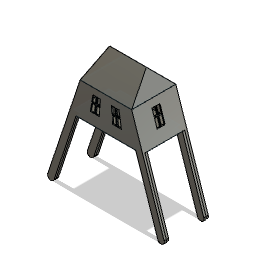
form10 v5 (Autodesk Fusion 360 design; units mm, degrees)
Autodesk Fusion 360 part; units mm, degrees
note: some values were not read from the file. Chosen so that the rebuilt part matches the saved one: which bodies a step acts on; which face or edge a step refers to. Set by a fixed rule: which sketch regions a step uses.
(part 1 of 2)
sketch "Sketch1" plane through (0, 0, 0) normal (0, 0, 1) x (1, 0, 0)
  line L0 (-100, 300) -> (100, 300)
  line L1 (100, 300) -> (100, 500)
  line L2 (100, 500) -> (-100, 500)
  line L3 (-100, 500) -> (-100, 300)
  line L4 (0, 0) -> (200, 0)
  line L5 (200, 0) -> (0, 0)
  line L6 (0, 0) -> (-200, 0)
  line L7 (-200, 0) -> (-100, 300)
  line L8 (100, 300) -> (200, 0)
  line L9 (-100, 500) -> (-266.666667, 0)
  line L10 (100, 500) -> (266.666667, 0)
  line L11 (163.504389, 309.486833) -> (135.04389, 300)
  line L12 (135.04389, 300) -> (100, 300)
  line L13 (-163.504389, 309.486833) -> (-135.04389, 300)
  line L14 (-135.04389, 300) -> (-100, 300)
  line L15 (-135.04389, 300) -> (-235.04389, 0)
  line L16 (135.04389, 300) -> (235.04389, 0)
  line L17 (266.666667, 0) -> (235.04389, 0)
  line L18 (-235.04389, 0) -> (-266.666667, 0)
  dimension "d1" = 200
  dimension "d2" = 200
  dimension "d3" = 30
  dimension "d4" = 30
  constraint horizontal L0
  constraint vertical L1
  constraint horizontal L2
  constraint vertical L3
  constraint coincident L4.start L5.end
  constraint perpendicular L3 L4
  constraint perpendicular L3 L6
  constraint parallel L7 L9
  constraint parallel L8 L10
  constraint perpendicular L10 L11
  constraint perpendicular L9 L13
  constraint parallel L9 L15
  constraint parallel L10 L16
  measures "d1" distance of L0.start L0.end
  measures "d2" distance of L0.start L2.end
extrude "Extrude1" add sketch "Sketch1" along normal blind 200 contours L0 L1 L2 L3 | L3 L9 L13 L14 | L1 L10 L11 L12 | L9 L13 L15 L18 | L10 L11 L16 L17 picked at (-33.333333, 433.333333) picked at (-121.16813, 369.828944) picked at (121.16813, 369.828944) picked at (-221.738315, 103.162278) picked at (221.738315, 103.162278) makes body 1
sketch "Sketch2" plane through (0, 0, 0) normal (1, 0, 0) x (0, 0, -1)
  line L0 (0, 500) -> (-200, 500)
  line L1 (-200, 500) -> (-200, 400)
  line L2 (-200, 400) -> (0, 400)
  line L3 (0, 400) -> (0, 500)
  line L4 (-100, 500) -> (0, 400)
  line L5 (-100, 500) -> (-200, 400)
  constraint horizontal L0
  constraint vertical L1
  constraint horizontal L2
  constraint vertical L3
  constraint midpoint L0 L4.start
  constraint perpendicular L4 L5
sketch "Sketch3" plane through (0, 500, 0) normal (0, 1, 0) x (-1, 0, 0)
  line L0 (-100, 0) -> (100, 0)
  line L1 (100, 0) -> (100, 200)
  line L2 (100, 200) -> (-100, 200)
  line L3 (-100, 200) -> (-100, 0)
sketch "Sketch4" plane through (0, 0, 0) normal (0, 0, -1) x (-1, 0, 0)
  line L0 (-135.04389, 300) -> (135.04389, 300)
  line L1 (135.04389, 300) -> (235.04389, 0)
  line L2 (235.04389, 0) -> (266.666667, 0)
  line L3 (266.666667, 0) -> (100, 500)
  line L4 (100, 500) -> (-100, 500)
  line L5 (-100, 500) -> (-266.666667, 0)
  line L6 (-266.666667, 0) -> (-235.04389, 0)
  line L7 (-235.04389, 0) -> (-135.04389, 300)
  line L8 (0, 500) -> (0, 550)
  line L9 (100, 550) -> (-100, 550)
  line L10 (100, 500) -> (83.333333, 550)
  line L11 (-100, 500) -> (-83.333333, 550)
  point P0 (0, 500)
  dimension "d7" = 50
  constraint coincident P0 L8.start
  constraint perpendicular L4 L8
  constraint horizontal L9
  constraint coincident L3.end L4.start
  constraint parallel L3 L10
  constraint coincident L4.end L5.start
  constraint parallel L5 L11
  measures "d7" distance of P0 L8.end
extrude "Extrude2" add sketch "Sketch4" against normal blind 200 contours L4 L8 L9 L11 | L4 L8 L9 L10 picked at (-61.111111, 516.666667) picked at (61.111111, 516.666667) bodies 1
sketch "Sketch5" plane through (0, 0, 0) normal (1, 0, 0) x (0, 0, -1)
  line L0 (-200, 550) -> (0, 550)
  line L1 (0, 550) -> (0, 450)
  line L2 (0, 450) -> (-200, 450)
  line L3 (-200, 450) -> (-200, 550)
  line L4 (-200, 550) -> (0, 550)
  line L5 (0, 550) -> (0, 500)
  line L6 (0, 500) -> (-200, 500)
  line L7 (-200, 500) -> (-200, 550)
  line L8 (-100, 550) -> (-200, 500)
  line L9 (0, 500) -> (-100, 550)
  line L10 (0, 450) -> (-100, 550)
  line L11 (-200, 450) -> (-100, 550)
  constraint horizontal L0
  constraint vertical L1
  constraint horizontal L2
  constraint vertical L3
  constraint horizontal L4
  constraint vertical L5
  constraint horizontal L6
  constraint vertical L7
  constraint midpoint L1 L5.end
  constraint midpoint L4 L8.start
  constraint perpendicular L10 L11
extrude "Extrude3" cut sketch "Sketch5" along normal blind 200 and the other way blind 200 contours L0 L3 L4 L7 L8 | L0 L1 L4 L5 L9 picked at (-166.666667, 533.333333) picked at (-33.333333, 533.333333) bodies 1
sketch "Sketch6" plane through (0, 0, 0) normal (1, 0, 0) x (0, 0, -1)
  line L0 (-20, 0) -> (-180, 0)
  line L1 (-180, 0) -> (-180, 300)
  line L2 (-180, 300) -> (-20, 300)
  line L3 (-20, 300) -> (-20, 0)
  dimension "d14" = 160
  dimension "d15" = 300
  constraint horizontal L0
  constraint vertical L1
  constraint horizontal L2
  constraint vertical L3
  measures "d14" distance of L0.start L0.end
  measures "d15" distance of L0.start L2.end
extrude "Extrude4" cut sketch "Sketch6" along normal blind 430 and the other way blind 320 bodies 1
sketch "Sketch7" plane through (0, 0, 0) normal (0, 0, -1) x (-1, 0, 0)
  line L0 (100, 500) -> (-100, 500)
  line L1 (-100, 500) -> (-266.666667, 0)
  line L2 (-266.666667, 0) -> (-235.04389, 0)
  line L3 (-235.04389, 0) -> (-135.04389, 300)
  line L4 (-135.04389, 300) -> (135.04389, 300)
  line L5 (135.04389, 300) -> (235.04389, 0)
  line L6 (235.04389, 0) -> (266.666667, 0)
  line L7 (266.666667, 0) -> (100, 500)
  line L8 (235.04389, 0) -> (263.504389, 9.486833)
  line L9 (249.27414, 4.743416) -> (240.606216, 30.747187)
  circle A0 centre (249.27414, 4.743416) radius 15
  line L10 (263.504389, 9.486833) -> (266.666667, 0)
  constraint perpendicular L7 L8
  constraint perpendicular L8 L9
extrude "Extrude5" cut sketch "Sketch7" against normal blind 300 contours L6 L7 A0 L10 picked at (264.700479, 0.516842) bodies 1
extrude "Extrude6" add sketch "Sketch7" against normal blind 20 separate body contours L6 L8 A0 | L8 L9 A0 | L8 L9 A0 | L6 A0 picked at (249.27414, 1.581139) picked at (248.203436, 14.660304) picked at (241.078294, 10.428413) picked at (245.376265, -2.550327) makes body 2
copy_body "CopyPasteBodies1" bodies 2 makes body 3
move_body "Move1" bodies 3 to x (1, 0, 0) y (0, 1, 0) z (0, 0, 1) at (0, 0, 180)
copy_body "CopyPasteBodies2" bodies 3 makes body 4
sketch "Sketch8" plane through (0, 0, 0) normal (0, 0, -1) x (-1, 0, 0)
  line L0 (-100, 500) -> (-266.666667, 0)
  line L1 (-235.04389, 0) -> (-263.504389, 9.486833)
  line L2 (-249.27414, 4.743416) -> (-238.791899, 36.190138)
  circle A0 centre (-249.27414, 4.743416) radius 15
  line L3 (-263.504389, 0) -> (-266.666667, 0)
  line L4 (-263.504389, 9.486833) -> (-266.666667, 0)
  point P0 (-235.04389, 0)
  constraint perpendicular L0 L1
  constraint perpendicular L1 L2
extrude "Extrude7" cut sketch "Sketch8" against normal blind 3000 contours L0 A0 L3 L4 picked at (-264.722183, 0.621872) bodies 1
extrude "Extrude8" add sketch "Sketch8" against normal blind 20 separate body contours L1 L2 A0 | L1 A0 | L1 L2 A0 picked at (-256.067662, 12.046781) picked at (-255.959942, -2.656664) picked at (-242.065982, 11.639917) makes body 5
copy_body "CopyPasteBodies3" bodies 5 makes body 6
move_body "Move2" bodies 6 to x (1, 0, 0) y (0, 1, 0) z (0, 0, 1) at (0, 0, 180)
extrude "Extrude9" cut sketch "Sketch5" along normal blind 225 and the other way blind 225 contours L0 L3 L4 L7 L8 | L6 L8 L11 | L0 L1 L4 L5 L9 | L6 L9 L10 | L3 L6 L11 | L1 L6 L10 picked at (-166.666667, 533.333333) picked at (-150, 516.666667) picked at (-33.333333, 533.333333) picked at (-50, 516.666667) picked at (-183.333333, 483.333333) picked at (-16.666667, 483.333333) bodies 1
sketch "Sketch9" plane through (0, 0, 200) normal (0, 0, 1) x (1, 0, 0)
  line L0 (116.666667, 450) -> (-116.666667, 450)
  line L1 (-116.666667, 450) -> (-263.504389, 9.486833)
  arc A0 (-263.504389, 9.486833) -> (-263.504389, 0) centre (-249.27414, 4.743416) ccw
  line L2 (-263.504389, 0) -> (-235.04389, 0)
  line L3 (-235.04389, 0) -> (-135.04389, 300)
  line L4 (-135.04389, 300) -> (135.04389, 300)
  line L5 (135.04389, 300) -> (235.04389, 0)
  line L6 (235.04389, 0) -> (263.504389, 0)
  arc A1 (263.504389, 0) -> (263.504389, 9.486833) centre (249.27414, 4.743416) ccw
  line L7 (263.504389, 9.486833) -> (116.666667, 450)
  line L8 (116.666667, 450) -> (-10.364311, 831.092932)
  line L9 (-116.666667, 450) -> (23.051535, 869.154604)
  line L10 (0, 800) -> (49.840939, -0.317043)
  line L11 (49.840939, -0.317043) -> (-46.807566, -0.317043)
  line L12 (-46.807566, -0.317043) -> (-150, -0.317043)
  line L13 (-150, -0.317043) -> (0, 800)
  line L14 (49.840939, -0.317043) -> (150, -0.317043)
  line L15 (150, -0.317043) -> (0, 800)
  line L16 (-50, -0.317043) -> (-50, -20)
  line L17 (49.840939, -0.317043) -> (-50, -0.317043)
  line L18 (-50, -0.317043) -> (0, 800)
  line L19 (-125, 325) -> (125, 325)
  line L20 (125, 325) -> (125, 425)
  line L21 (125, 425) -> (-125, 425)
  line L22 (-125, 425) -> (-125, 325)
  line L23 (-125, 375) -> (125, 375)
  line L24 (-98.403783, -0.317043) -> (0, 800)
  line L25 (99.92047, -0.317043) -> (0, 800)
  line L26 (-100.388834, -0.072969) -> (-0.015179, 816.265027)
  line L27 (101.905062, -0.069264) -> (-0.015179, 816.265027)
  line L28 (-96.418732, -0.561117) -> (0.015179, 783.734974)
  line L29 (97.935878, -0.564821) -> (0.015179, 783.734974)
  line L30 (-125, 373) -> (125, 373)
  line L31 (-125, 377) -> (125, 377)
  line L32 (-145.180647, 3.682957) -> (0, 778.286596)
  line L33 (145.180647, 3.682957) -> (0, 778.286596)
  line L34 (49.840939, 3.682957) -> (145.180647, 3.682957)
  line L35 (49.840939, 3.682957) -> (-46.807566, 3.682957)
  line L36 (-46.807566, 3.682957) -> (-145.180647, 3.682957)
  line L37 (-53.992216, -0.067628) -> (0.00636, 864.251996)
  line L38 (0.00636, 864.251996) -> (53.833205, -0.068418)
  line L39 (-121, 329) -> (121, 329)
  line L40 (121, 329) -> (121, 421)
  line L41 (121, 421) -> (-121, 421)
  line L42 (-121, 421) -> (-121, 329)
  line L43 (116.666667, 450, 0) -> (116.666667, 450, -200)
  line L44 (-116.666667, 450, 0) -> (-116.666667, 450, -200)
  line L45 (-170, 300) -> (170, 300)
  line L46 (170, 300) -> (170, 450)
  line L47 (170, 450) -> (-170, 450)
  line L48 (-170, 450) -> (-170, 300)
  line L49 (0, 300) -> (167.029465, 300)
  line L50 (167.029465, 300) -> (167.029465, 450)
  line L51 (167.029465, 450) -> (0, 450)
  line L52 (0, 450) -> (0, 300)
  point P0 (116.666667, 450)
  point P1 (-116.666667, 450)
  dimension "d32" = 2
  dimension "d33" = -2
  dimension "d34" = 2
  dimension "d35" = -2
  dimension "d36" = 4
  dimension "d37" = -4
  dimension "d38" = -4
  constraint parallel L7 L8
  constraint parallel L1 L9
  constraint coincident L8 L10.start
  constraint coincident L9 L10.start
  constraint horizontal L11
  constraint parallel L11 L12
  constraint parallel L11 L14
  constraint horizontal L19
  constraint vertical L20
  constraint horizontal L21
  constraint vertical L22
  constraint coincident L7 L20.end
  constraint midpoint L22 L23.start
  constraint midpoint L20 L23.end
  constraint horizontal L45
  constraint vertical L46
  constraint horizontal L47
  constraint vertical L48
  constraint horizontal L49
  constraint vertical L50
  constraint horizontal L51
  constraint vertical L52
sketch "Sketch10" plane through (0, 0, 200) normal (0, 0, 1) x (1, 0, 0)
  line L0 (0, 300) -> (-166.775998, 300)
  line L1 (-166.775998, 300) -> (-166.775998, 450.114505)
  line L2 (0, 450.114505) -> (0, 300)
  line L3 (116.666667, 450) -> (83.333333, 550)
  line L4 (83.333333, 550) -> (-18.03309, 854.099269)
  line L5 (-116.666667, 450) -> (-83.333333, 550)
  line L6 (-83.333333, 550) -> (27.18713, 881.561391)
  line L7 (30, 350) -> (70, 350)
  line L8 (-30, 350) -> (-70, 350)
  line L9 (-70, 350) -> (0, 800)
  line L10 (70, 350) -> (0, 800)
  line L11 (30, 350) -> (0, 800)
  line L12 (-30, 350) -> (0, 800)
  line L13 (59.111111, 420) -> (-59.111111, 420)
  line L14 (50, 350) -> (0, 800)
  line L15 (-50, 350) -> (0, 800)
  line L16 (-25.333333, 420) -> (-70, 350)
  line L17 (-59.111111, 420) -> (-30, 350)
  line L18 (59.111111, 420) -> (30, 350)
  line L19 (25.333333, 420) -> (70, 350)
  line L20 (45.783133, 387.951807) -> (-45.783133, 387.951807)
  line L21 (45.783133, 387.951807) -> (64.096386, 387.951807)
  line L22 (-45.783133, 387.951807) -> (-64.096386, 387.951807)
  line L23 (-45.783133, 389.951807) -> (-64.096386, 389.951807)
  line L24 (45.783133, 389.951807) -> (-45.783133, 389.951807)
  line L25 (45.783133, 389.951807) -> (64.096386, 389.951807)
  line L26 (-45.783133, 385.951807) -> (-64.096386, 385.951807)
  line L27 (45.783133, 385.951807) -> (-45.783133, 385.951807)
  line L28 (45.783133, 385.951807) -> (64.096386, 385.951807)
  line L29 (-51.987767, 350.220863) -> (0, 818.11077)
  line L30 (51.987767, 350.220863) -> (0, 818.11077)
  line L31 (-48.012233, 349.779137) -> (0, 781.88923)
  line L32 (48.012233, 349.779137) -> (0, 781.88923)
  line L33 (-51.987767, 350.220863) -> (-53.194502, 339.36025)
  line L34 (51.987767, 350.220863) -> (53.06275, 340.546021)
  line L35 (-64.096386, 385.951807) -> (-76.613224, 385.951807)
  line L36 (64.096386, 385.951807) -> (88.42743, 385.951807)
  point P0 (-83.333333, 550)
  point P1 (-116.666667, 450)
  point P2 (116.666667, 450)
  point P3 (83.333333, 550)
  dimension "d40" = 2
  dimension "d41" = -2
  dimension "d42" = 2
  dimension "d43" = -2
  constraint horizontal L0
  constraint vertical L1
  constraint vertical L2
  constraint parallel L3 L4
  constraint parallel L5 L6
  constraint horizontal L7
  constraint horizontal L8
  constraint coincident L6 L9.end
  constraint coincident L4 L9.end
  constraint midpoint L7 L14.start
  constraint midpoint L8 L15.start
  constraint horizontal L21
  constraint parallel L20 L22
  constraint parallel L29 L33
  constraint parallel L30 L34
  constraint parallel L26 L35
  constraint parallel L28 L36
extrude "Extrude10" cut sketch "Sketch10" against normal blind 340 contours L11 L19 L24 L32 | L13 L19 L32 | L13 L16 L31 | L12 L16 L24 L31 | L11 L18 L27 L32 | L12 L17 L27 L31 | L13 L18 L30 | L13 L17 L29 | L7 L18 L32 | L8 L17 L31 | L9 L17 L23 L29 | L10 L18 L25 L30 | L10 L19 L28 L30 L36 | L7 L19 L30 L34 | L8 L16 L29 L33 | L9 L16 L26 L29 L35 picked at (32.005474, 400.57405) picked at (36.296597, 410.590114) picked at (-36.296597, 410.590114) picked at (-32.005474, 400.57405) picked at (33.932773, 373.361693) picked at (-33.932773, 373.361693) picked at (50.238933, 410.590114) picked at (-50.238933, 410.590114) picked at (40.7276, 361.377757) picked at (-40.7276, 361.377757) picked at (-56.755848, 400.57405) picked at (56.755848, 400.57405) picked at (60.772036, 373.361693) picked at (56.73583, 361.451378) picked at (-56.73583, 361.451378) picked at (-60.772036, 373.361693) bodies 1
sketch "Sketch11" plane through (0, 0, 0) normal (1, 0, 0) x (0, 0, -1)
sketch "Sketch12" plane through (0, 0, 0) normal (1, 0, 0) x (0, 0, -1)
  line L0 (-105, 420) -> (-85, 420)
  line L1 (-85, 420) -> (-85, 350.000005)
  line L2 (-85, 350.000005) -> (-105, 350.000005)
  line L3 (-105, 350.000005) -> (-105, 420)
  line L4 (-105, 420) -> (-125, 420)
  line L5 (-125, 420) -> (-125, 350)
  line L6 (-125, 350) -> (-105, 350)
  line L7 (-105, 350) -> (-105, 420)
  line L8 (-103, 418) -> (-87, 418)
  line L9 (-87, 418) -> (-87, 352.000005)
  line L10 (-87, 352.000005) -> (-103, 352.000005)
  line L11 (-103, 352.000005) -> (-103, 418)
  line L12 (-107, 418) -> (-123, 418)
  line L13 (-123, 418) -> (-123, 352)
  line L14 (-123, 352) -> (-107, 352)
  line L15 (-107, 352) -> (-107, 418)
  line L16 (-107, 420) -> (-107, 350)
  line L17 (-103, 420) -> (-103, 350)
  line L18 (-87, 420) -> (-87, 350)
  line L19 (-123, 420) -> (-123, 350)
  line L20 (-85, 390) -> (-125, 390)
  line L21 (-125, 386.000006) -> (-85, 386.000006)
  dimension "d46" = 20
  dimension "d47" = 70
  dimension "d48" = 2
  dimension "d49" = -2
  constraint horizontal L0
  constraint vertical L1
  constraint horizontal L2
  constraint vertical L3
  constraint horizontal L4
  constraint vertical L5
  constraint horizontal L6
  constraint vertical L7
  constraint coincident L4 L16.start
  constraint coincident L6 L16.end
  constraint perpendicular L6 L16
  constraint coincident L0 L17.start
  constraint coincident L2 L17.end
  constraint perpendicular L2 L17
  constraint coincident L0 L18.start
  constraint coincident L2 L18.end
  constraint perpendicular L2 L18
  constraint coincident L4 L19.start
  constraint coincident L6 L19.end
  constraint perpendicular L6 L19
  constraint coincident L1 L20.start
  constraint coincident L5 L20.end
  constraint perpendicular L5 L20
  constraint perpendicular L1 L21
  measures "d46" distance of L0.start L0.end
  measures "d47" distance of L0.start L6.end
extrude "Extrude11" cut sketch "Sketch12" along normal blind 310 and the other way blind 250 contours L0 L8 L17 L18 | L4 L12 L16 L19 | L8 L9 L11 L17 L18 L20 | L12 L13 L15 L16 L19 L20 | L13 L14 L15 L16 L19 L21 | L9 L10 L11 L17 L18 L21 | L2 L10 L17 L18 | L6 L14 L16 L19 picked at (-97.666667, 418.666667) picked at (-117.666667, 418.666667) picked at (-97.666667, 408.666667) picked at (-117.666667, 408.666667) picked at (-112.333333, 363.333335) picked at (-97.666667, 363.333339) picked at (-92.333333, 351.333339) picked at (-117.666667, 350.666668) bodies 1
sketch "Sketch13" plane through (0, 0, 200) normal (0, 0, 1) x (1, 0, 0)
  line L0 (27.336546, 389.951807) -> (25.333333, 420)
  line L1 (25.333333, 420) -> (40.209914, 420)
  line L2 (40.209914, 420) -> (43.548602, 389.951807)
  line L3 (43.548602, 389.951807) -> (27.336546, 389.951807)
  line L4 (-63.785274, 389.951807) -> (-59.111111, 420)
  line L5 (-59.111111, 420) -> (-44.23453, 420)
  line L6 (-44.23453, 420) -> (-47.573218, 389.951807)
  line L7 (-47.573218, 389.951807) -> (-63.785274, 389.951807)
  line L8 (-64.407497, 385.951807) -> (-48.017663, 385.951807)
  line L9 (-48.017663, 385.951807) -> (-52.012308, 350)
  line L10 (-52.012308, 350) -> (-70, 350)
  line L11 (-70, 350) -> (-64.407497, 385.951807)
  line L12 (59.111111, 420) -> (63.785274, 389.951807)
  line L13 (63.785274, 389.951807) -> (47.573218, 389.951807)
  line L14 (47.573218, 389.951807) -> (44.23453, 420)
  line L15 (44.23453, 420) -> (59.111111, 420)
  line L16 (43.993047, 385.951807) -> (47.987692, 350)
  line L17 (47.987692, 350) -> (30, 350)
  line L18 (30, 350) -> (27.603213, 385.951807)
  line L19 (27.603213, 385.951807) -> (43.993047, 385.951807)
  line L20 (-43.548602, 389.951807) -> (-40.209914, 420)
  line L21 (-40.209914, 420) -> (-25.333333, 420)
  line L22 (-25.333333, 420) -> (-27.336546, 389.951807)
  line L23 (-27.336546, 389.951807) -> (-43.548602, 389.951807)
  line L24 (-47.987692, 350) -> (-43.993047, 385.951807)
  line L25 (-43.993047, 385.951807) -> (-27.603213, 385.951807)
  line L26 (-27.603213, 385.951807) -> (-30, 350)
  line L27 (-30, 350) -> (-47.987692, 350)
  line L28 (70, 350) -> (52.012308, 350)
  line L29 (52.012308, 350) -> (48.017663, 385.951807)
  line L30 (48.017663, 385.951807) -> (64.407497, 385.951807)
  line L31 (64.407497, 385.951807) -> (70, 350)
  line L32 (116.666667, 450) -> (-116.666667, 450)
  line L33 (-116.666667, 450) -> (-263.504389, 9.486833)
  arc A0 (-263.504389, 9.486833) -> (-263.504389, 0) centre (-249.27414, 4.743416) ccw
  line L34 (-263.504389, 0) -> (-235.04389, 0)
  line L35 (-235.04389, 0) -> (-135.04389, 300)
  line L36 (-135.04389, 300) -> (135.04389, 300)
  line L37 (135.04389, 300) -> (235.04389, 0)
  line L38 (235.04389, 0) -> (263.504389, 0)
  arc A1 (263.504389, 0) -> (263.504389, 9.486833) centre (249.27414, 4.743416) ccw
  line L39 (263.504389, 9.486833) -> (116.666667, 450)
  line L40 (200, 450) -> (-200, 450)
  line L41 (-200, 450) -> (-200, 602.828066)
  line L42 (-200, 602.828066) -> (200, 602.828066)
  line L43 (200, 602.828066) -> (200, 450)
  dimension "d54" = 400
  constraint horizontal L40
  constraint vertical L41
  constraint horizontal L42
  constraint vertical L43
  measures "d54" distance of L40.start L40.end
split "Split1" by curves path "Sketch13" along L42 L43 L40 L41 bodies 1 makes body 7 at (-45.01463, 300, 73.333333)
sketch "Sketch14" plane through (0, 325, 325) normal (0, 0.707107, 0.707107) x (1, 0, 0)
  line L0 (116.666667, 176.776695) -> (83.333333, 318.198052)
  line L1 (83.333333, 318.198052) -> (-83.333333, 318.198052)
  line L2 (-83.333333, 318.198052) -> (-116.666667, 176.776695)
  line L3 (-116.666667, 176.776695) -> (116.666667, 176.776695)
  line L4 (-79.374833, 313.198052) -> (-110.351144, 181.776695)
  line L5 (-110.351144, 181.776695) -> (110.351144, 181.776695)
  line L6 (110.351144, 181.776695) -> (79.374833, 313.198052)
  line L7 (79.374833, 313.198052) -> (-79.374833, 313.198052)
  dimension "d55" = -5
extrude "Extrude12" cut sketch "Sketch14" along normal blind -240 and the other way blind 5 contours L4 L5 L6 L7 picked at (-26.458278, 225.583814) bodies 1
sketch "Sketch15" plane through (0, 225, -225) normal (0, 0.707107, -0.707107) x (-1, 0, 0)
  line L0 (-83.333333, 459.619408) -> (-116.666667, 318.198052)
  line L1 (-116.666667, 318.198052) -> (116.666667, 318.198052)
  line L2 (116.666667, 318.198052) -> (83.333333, 459.619408)
  line L3 (83.333333, 459.619408) -> (-83.333333, 459.619408)
  line L4 (110.351144, 323.198052) -> (79.374833, 454.619408)
  line L5 (79.374833, 454.619408) -> (-79.374833, 454.619408)
  line L6 (-79.374833, 454.619408) -> (-110.351144, 323.198052)
  line L7 (-110.351144, 323.198052) -> (110.351144, 323.198052)
  dimension "d60" = -5
extrude "Extrude13" cut sketch "Sketch15" along normal blind -180 and the other way blind 5 contours L4 L5 L6 L7 picked at (26.458278, 367.00517) bodies 1
sketch "Sketch16" plane through (-240, 80, 0) normal (-0.948683, 0.316228, 0) x (0, 0, 1)
  line L0 (0, 390.014245) -> (200, 390.014245)
  line L1 (200, 390.014245) -> (100, 495.4235)
  line L2 (100, 495.4235) -> (0, 390.014245)
  line L3 (11.635441, 395.014245) -> (188.364559, 395.014245)
  line L4 (188.364559, 395.014245) -> (100, 488.158669)
  line L5 (100, 488.158669) -> (11.635441, 395.014245)
  line L6 (11.635441, 395.014245) -> (-12.394431, 369.684536)
  line L7 (188.364559, 395.014245) -> (205.575241, 376.872594)
  dimension "d65" = -5
  constraint parallel L5 L6
  constraint parallel L4 L7
extrude "Extrude14" cut sketch "Sketch16" along normal blind -40 and the other way blind 6 contours L0 L3 L6 L7 | L3 L4 L5 picked at (129.454853, 391.680911) picked at (100, 426.062386) bodies 1
sketch "Sketch17" plane through (240, 80, 0) normal (0.948683, 0.316228, 0) x (0, 0, -1)
  line L0 (-200, 390.014245) -> (0, 390.014245)
  line L1 (0, 390.014245) -> (-100, 495.4235)
  line L2 (-100, 495.4235) -> (-200, 390.014245)
  line L3 (-100, 490) -> (-7, 392.000006)
  line L4 (-7, 392.000006) -> (-0.785722, 386.104624)
  line L5 (-100, 490) -> (-193.000003, 392.000006)
  line L6 (-193.000003, 392.000006) -> (-201.192859, 383.366675)
  constraint perpendicular L2 L4
  constraint parallel L5 L6
extrude "Extrude15" cut sketch "Sketch17" along normal blind -50 and the other way blind 6 contours L0 L3 L4 L5 L6 picked at (-100.000001, 424.666671) bodies 1
sketch "Sketch18" plane through (-240, 80, 0) normal (-0.948683, 0.316228, 0) x (0, 0, 1)
  line L0 (0, 390.014245) -> (200, 390.014245)
  line L1 (200, 390.014245) -> (100, 495.4235)
  line L2 (100, 495.4235) -> (0, 390.014245)
  line L3 (100, 490) -> (7.077367, 392.050945)
  line L4 (7.077367, 392.050945) -> (-0.940246, 383.599639)
  line L5 (100, 490) -> (196.278995, 388.513028)
  line L6 (196.278995, 388.513028) -> (-0.940246, 383.599639)
  constraint parallel L2 L3
  constraint parallel L1 L5
extrude "Extrude16" cut sketch "Sketch18" along normal blind -40 and the other way blind 6 contours L0 L3 L4 L5 picked at (100.644061, 424.02173) bodies 1
sketch "Sketch19" plane through (0, 0, 0) normal (0, 0, -1) x (-1, 0, 0)
  line L0 (-25.333333, 420) -> (-27.336546, 389.951807)
  line L1 (-27.336546, 389.951807) -> (-43.548602, 389.951807)
  line L2 (-43.548602, 389.951807) -> (-40.209914, 420)
  line L3 (-40.209914, 420) -> (-25.333333, 420)
  line L4 (59.111111, 420) -> (63.785274, 389.951807)
  line L5 (63.785274, 389.951807) -> (47.573218, 389.951807)
  line L6 (47.573218, 389.951807) -> (44.23453, 420)
  line L7 (44.23453, 420) -> (59.111111, 420)
  line L8 (48.017663, 385.951807) -> (64.407497, 385.951807)
  line L9 (64.407497, 385.951807) -> (70, 350)
  line L10 (70, 350) -> (52.012308, 350)
  line L11 (52.012308, 350) -> (48.017663, 385.951807)
  line L12 (-63.785274, 389.951807) -> (-59.111111, 420)
  line L13 (-59.111111, 420) -> (-44.23453, 420)
  line L14 (-44.23453, 420) -> (-47.573218, 389.951807)
  line L15 (-47.573218, 389.951807) -> (-63.785274, 389.951807)
  line L16 (-47.987692, 350) -> (-43.993047, 385.951807)
  line L17 (-43.993047, 385.951807) -> (-27.603213, 385.951807)
  line L18 (-27.603213, 385.951807) -> (-30, 350)
  line L19 (-30, 350) -> (-47.987692, 350)
  line L20 (40.209914, 420) -> (43.548602, 389.951807)
  line L21 (43.548602, 389.951807) -> (27.336546, 389.951807)
  line L22 (27.336546, 389.951807) -> (25.333333, 420)
  line L23 (25.333333, 420) -> (40.209914, 420)
  line L24 (43.993047, 385.951807) -> (47.987692, 350)
  line L25 (47.987692, 350) -> (30, 350)
  line L26 (30, 350) -> (27.603213, 385.951807)
  line L27 (27.603213, 385.951807) -> (43.993047, 385.951807)
  line L28 (-52.012308, 350) -> (-70, 350)
  line L29 (-70, 350) -> (-64.407497, 385.951807)
  line L30 (-64.407497, 385.951807) -> (-48.017663, 385.951807)
  line L31 (-48.017663, 385.951807) -> (-52.012308, 350)
  line L32 (116.666667, 450) -> (-116.666667, 450)
  line L33 (-116.666667, 450) -> (-263.504389, 9.486833)
  arc A0 (-263.504389, 9.486833) -> (-263.504389, 0) centre (-249.27414, 4.743416) ccw
  line L34 (-263.504389, 0) -> (-235.04389, 0)
  line L35 (-235.04389, 0) -> (-135.04389, 300)
  line L36 (-135.04389, 300) -> (135.04389, 300)
  line L37 (135.04389, 300) -> (235.04389, 0)
  line L38 (235.04389, 0) -> (263.504389, 0)
  arc A1 (263.504389, 0) -> (263.504389, 9.486833) centre (249.27414, 4.743416) ccw
  line L39 (263.504389, 9.486833) -> (116.666667, 450)
  line L40 (-116.666667, 450) -> (-166.778531, 299.664408)
  line L41 (166.778531, 299.664408) -> (116.666667, 450)
  arc A2 (-258.760973, 7.905694) -> (-259.270847, 5) centre (-249.27414, 4.743416) ccw
  line L42 (-259.270847, 5) -> (-238.647686, 5)
  line L43 (-238.647686, 5) -> (-138.647686, 305)
  line L44 (-138.647686, 305) -> (138.647686, 305)
  line L45 (138.647686, 305) -> (238.647686, 5)
  line L46 (238.647686, 5) -> (259.270847, 5)
  arc A3 (259.270847, 5) -> (258.760973, 7.905694) centre (249.27414, 4.743416) ccw
  line L47 (258.760973, 7.905694) -> (113.062871, 445)
  line L48 (113.062871, 445) -> (-113.062871, 445)
  line L49 (-113.062871, 445) -> (-258.760973, 7.905694)
  line L50 (-138.647686, 305) -> (-176.025835, 305)
  line L51 (-176.025835, 305) -> (138.647686, 305)
  line L52 (210, 305) -> (138.647686, 305)
  dimension "d78" = -5
  constraint parallel L33 L40
  constraint parallel L39 L41
  constraint parallel L44 L50
  constraint parallel L51 L52
extrude "Extrude17" cut sketch "Sketch19" along normal blind -195 and the other way blind 5 contours L44 L47 L48 L49 L50 L51 L52 picked at (107.236852, 366.666667) bodies 7
sketch "Sketch20" plane through (0, 450, 0) normal (0, 1, 0) x (-1, 0, 0)
  line L0 (-116.666667, 0) -> (116.666667, 0)
  line L1 (116.666667, 0) -> (116.666667, 200)
  line L2 (116.666667, 200) -> (-116.666667, 200)
  line L3 (-116.666667, 200) -> (-116.666667, 0)
  line L4 (111.666667, 195) -> (-111.666667, 195)
  line L5 (-111.666667, 195) -> (-111.666667, 5)
  line L6 (-111.666667, 5) -> (111.666667, 5)
  line L7 (111.666667, 5) -> (111.666667, 195)
  dimension "d83" = -5
extrude "Extrude18" cut sketch "Sketch20" against normal blind 40 contours L4 L5 L6 L7 picked at (37.222222, 68.333333) bodies 7
sketch "Sketch21" plane through (0, 450, 0) normal (0, 1, 0) x (-1, 0, 0)
  line L0 (-111.666667, 195) -> (111.666667, 195)
  line L1 (111.666667, 195) -> (111.666667, 5)
  line L2 (111.666667, 5) -> (-111.666667, 5)
  line L3 (-111.666667, 5) -> (-111.666667, 195)
  line L4 (-116.666667, 0) -> (116.666667, 0)
  line L5 (116.666667, 0) -> (116.666667, 200)
  line L6 (116.666667, 200) -> (-116.666667, 200)
  line L7 (-116.666667, 200) -> (-116.666667, 0)
sketch "Sketch22" plane through (0, 450, 0) normal (0, 1, 0) x (-1, 0, 0)
  line L0 (-110.666667, 6) -> (110.666667, 6)
  line L1 (110.666667, 6) -> (110.666667, 194)
  line L2 (110.666667, 194) -> (-110.666667, 194)
  line L3 (-110.666667, 194) -> (-110.666667, 6)
  line L4 (-105.666667, 189) -> (-105.666667, 11)
  line L5 (-105.666667, 11) -> (105.666667, 11)
  line L6 (105.666667, 11) -> (105.666667, 189)
  line L7 (105.666667, 189) -> (-105.666667, 189)
  point P0 (-110.666667, 6)
  point P1 (110.666667, 194)
  dimension "d87" = -5
  constraint horizontal L0
  constraint vertical L1
  constraint horizontal L2
  constraint vertical L3
extrude "Extrude19" add sketch "Sketch22" along normal blind 2 and the other way blind 4 bodies 1
sketch "Sketch23" plane through (0, 300, 0) normal (0, -1, 0) x (1, 0, 0)
  line L0 (135.04389, 180) -> (135.04389, 200)
  line L1 (135.04389, 200) -> (-135.04389, 200)
  line L2 (-135.04389, 200) -> (-135.04389, 180)
  line L3 (-135.04389, 180) -> (-166.666667, 180)
  line L4 (-166.666667, 180) -> (-166.666667, 20)
  line L5 (-166.666667, 20) -> (-135.04389, 20)
  line L6 (-135.04389, 20) -> (-135.04389, 0)
  line L7 (-135.04389, 0) -> (135.04389, 0)
  line L8 (135.04389, 0) -> (135.04389, 20)
  line L9 (135.04389, 20) -> (166.666667, 20)
  line L10 (166.666667, 20) -> (166.666667, 180)
  line L11 (166.666667, 180) -> (135.04389, 180)
sketch "Sketch24" plane through (0, 0, 0) normal (0, 1, 0) x (1, 0, 0)
  circle A0 centre (0, -100) radius 15
  dimension "d92" = 30
  measures "d92" diameter of A0
extrude "Extrude20" cut sketch "Sketch24" along normal blind 340 bodies 7
sketch "Sketch25" plane through (0, 450, 0) normal (0, 1, 0) x (-1, 0, 0)
  line L0 (0, 100) -> (0, 130)
  line L1 (0, 100) -> (0, 70)
  line L2 (-15, 100) -> (-20, 100)
  line L3 (-20, 100) -> (-20, 130)
  line L4 (-20, 100) -> (120, 100)
  line L5 (-20, 130) -> (120, 130)
  line L6 (120, 130) -> (120, 70)
  line L7 (120, 70) -> (-20, 70)
  line L8 (-20, 70) -> (-20, 130)
  dimension "d95" = 30
  dimension "d96" = 30
  dimension "d97" = 5
  dimension "d98" = 140
  dimension "d99" = 140
  dimension "d100" = 60
  constraint vertical L0
  constraint parallel L0 L1
  constraint perpendicular L1 L2
  constraint perpendicular L2 L3
  constraint perpendicular L3 L4
  constraint horizontal L5
  constraint vertical L6
  constraint horizontal L7
  constraint vertical L8
  measures "d95" distance of L0.start L0.end
  measures "d96" distance of L0.start L1.end
  measures "d97" distance of L2.start L2.end
  measures "d98" distance of L2.end L4.end
  measures "d99" distance of L3.end L5.end
  measures "d100" distance of L3.end L7.end
extrude "Extrude21" add sketch "Sketch25" along normal blind 100 separate body makes body 8
move_body "Move3" bodies 8 to x (1, 0, 0) y (0, 1, 0) z (0, 0, 1) at (0, -130, 0)
sketch "Sketch26" plane through (0, 300, 0) normal (0, -1, 0) x (1, 0, 0)
  circle A0 centre (0, 100.000001) radius 12.5
  dimension "d106" = 25
  measures "d106" diameter of A0
extrude "Extrude22" add sketch "Sketch26" against normal blind 26 bodies 8
sketch "Sketch27" plane through (0, 300, 0) normal (0, -1, 0) x (1, 0, 0)
  circle A0 centre (0, 100) radius 20
  circle A1 centre (0, 100) radius 15
  dimension "d110" = 40
  constraint concentric A0 A1
  measures "d110" diameter of A0
extrude "Extrude23" cut sketch "Sketch27" against normal blind 20 contours A0 | A1 picked at (18.203026, 98.261174) picked at (-0.398504, 104.654369) bodies 7 8
move_body "Move4" bodies 8 to x (1, 0, 0) y (0, 1, 0) z (0, 0, 1) at (5, 0, 0)
sketch "Sketch28" plane through (0, 300, 0) normal (0, -1, 0) x (1, 0, 0)
  circle A0 centre (0, 100) radius 17.5
  circle A1 centre (0, 100) radius 20
  dimension "d116" = 35
  constraint concentric A0 A1
  measures "d116" diameter of A0
extrude "Extrude24" add sketch "Sketch28" against normal blind 25 contours A0 picked at (4.88488, 104.155447) bodies 8
sketch "Sketch29" plane through (0, 300, 0) normal (0, -1, 0) x (1, 0, 0)
  line L0 (24.948091, 100) -> (34.948091, 100)
  line L1 (34.948091, 100) -> (34.948091, 105)
  line L2 (34.948091, 105) -> (24.948091, 105)
  line L3 (24.948091, 105) -> (24.948091, 100)
  line L4 (24.948091, 100) -> (34.948091, 100)
  line L5 (34.948091, 100) -> (34.948091, 95)
  line L6 (34.948091, 95) -> (24.948091, 95)
  line L7 (24.948091, 95) -> (24.948091, 100)
  dimension "d119" = 10
  dimension "d120" = 5
  dimension "d121" = 5
  constraint horizontal L0
  constraint vertical L1
  constraint horizontal L2
  constraint vertical L3
  constraint horizontal L4
  constraint vertical L5
  constraint horizontal L6
  constraint vertical L7
extrude "Extrude25" cut sketch "Sketch29" against normal blind 10 bodies 7
move_face "MoveFace1" by (0, 0, -5) 32 faces at (-64.004103, 350, 3.333333) (-133.153025, 390, 92.333333) (-144.243178, 362.000002, 87) (138.486357, 374.000004, 103) (136.243177, 386.000006, 117.666667) (-144.243178, 362.000002, 123) (-133.153025, 390, 112.333333) (126.486358, 410, 123) (138.486357, 374.000004, 87) (-126.486358, 410, 123) (-144.243178, 362.000002, 103) (146.486358, 350.000005, 92.333333) (-123.153025, 420, 117.666667) (134.909846, 390, 112.333333) (-123.153025, 420, 92.333333) (-138.486357, 374.000004, 107) (126.486358, 410, 107) (124.909846, 420, 112.333333) (126.486358, 410, 87) (134.909846, 390, 92.333333) (-134.486356, 386.000006, 112.333333) (123.153025, 420, 97.666667) (-126.486358, 410, 103) (138.486357, 374.000004, 107) (-126.486358, 410, 107) (-64.004103, 350, 196.666667) (-126.486358, 410, 87) (144.243178, 362.000002, 123) (-35.995897, 350, 1.666667) (-146.486358, 350.000005, 92.333333) (126.486358, 410, 103) (-35.995897, 350, 196.666667) on bodies 7
sketch "Sketch30" plane through (0, 300, 0) normal (0, -1, 0) x (1, 0, 0)
  line L0 (25, 95) -> (55, 95)
  line L1 (55, 95) -> (55, 115)
  line L2 (55, 115) -> (25, 115)
  line L3 (25, 115) -> (25, 95)
  line L4 (55, 95) -> (25, 95)
  line L5 (25, 95) -> (25, 85)
  line L6 (25, 85) -> (55, 85)
  line L7 (55, 85) -> (55, 95)
  line L8 (35, 115) -> (65, 115)
  line L9 (65, 115) -> (65, 85)
  line L10 (65, 85) -> (35, 85)
  line L11 (35, 85) -> (35, 115)
  dimension "d124" = 30
  dimension "d125" = 30
  dimension "d126" = 10
  dimension "d127" = 30
  dimension "d128" = 30
  constraint horizontal L0
  constraint vertical L1
  constraint horizontal L2
  constraint vertical L3
  constraint horizontal L4
  constraint vertical L5
  constraint horizontal L6
  constraint vertical L7
  constraint horizontal L8
  constraint vertical L9
  constraint horizontal L10
  constraint vertical L11
  constraint coincident L2 L8.start
  measures "d124" distance of L0.start L0.end
  measures "d125" distance of L0.end L0.start
  measures "d126" distance of L0.end L6.end
  measures "d127" distance of L8.start L8.end
  measures "d128" distance of L8.start L10.end
extrude "Extrude26" cut sketch "Sketch30" against normal blind 10 contours L0 L2 L3 L4 L11 | L0 L4 L5 L6 L11 | L0 L1 L2 L4 L8 L11 | L0 L4 L6 L7 L10 L11 picked at (28.333333, 108.333333) picked at (28.333333, 91.666667) picked at (41.666667, 108.333333) picked at (41.666667, 91.666667) bodies 7
sketch "Sketch31" plane through (0, 300, 0) normal (0, -1, 0) x (1, 0, 0)
  line L0 (-40, 120) -> (-42, 120)
  line L1 (-42, 120) -> (-42, 80)
  line L2 (-42, 80) -> (-40, 80)
  line L3 (-40, 80) -> (-40, 120)
  line L4 (-42, 120) -> (-44, 120)
  line L5 (-44, 120) -> (-44, 80)
  line L6 (-44, 80) -> (-42, 80)
  line L7 (-42, 80) -> (-42, 120)
  line L8 (-44, 120) -> (-46, 120)
  line L9 (-46, 120) -> (-46, 80)
  line L10 (-46, 80) -> (-44, 80)
  line L11 (-44, 80) -> (-44, 120)
  line L12 (-46, 120) -> (-48, 120)
  line L13 (-48, 120) -> (-48, 80)
  line L14 (-48, 80) -> (-46, 80)
  line L15 (-46, 80) -> (-46, 120)
  line L16 (-50, 120) -> (-50, 80)
  line L17 (-50, 120) -> (-52, 120)
  line L18 (-52, 120) -> (-52, 80)
  line L19 (-52, 80) -> (-50, 80)
  line L20 (-50, 80) -> (-50, 120)
  line L21 (-48, 120) -> (-50, 120)
  line L22 (-50, 120) -> (-50, 80)
  line L23 (-50, 80) -> (-48, 80)
  line L24 (-48, 80) -> (-48, 120)
  line L25 (-58, 80) -> (-58, 120)
  line L26 (-64, 80) -> (-64, 120)
  line L27 (-60, 80) -> (-60, 120)
  line L28 (-56, 80) -> (-56, 120)
  line L29 (-64, 120) -> (-64, 80)
  line L30 (-54, 120) -> (-56, 120)
  line L31 (-56, 120) -> (-58, 120)
  line L32 (-60, 120) -> (-62, 120)
  line L33 (-66, 120) -> (-66, 80)
  line L34 (-54, 80) -> (-54, 120)
  line L35 (-64, 120) -> (-66, 120)
  line L36 (-66, 80) -> (-64, 80)
  line L37 (-56, 80) -> (-54, 80)
  line L38 (-58, 80) -> (-56, 80)
  line L39 (-60, 80) -> (-58, 80)
  line L40 (-58, 120) -> (-58, 80)
  line L41 (-62, 120) -> (-62, 80)
  line L42 (-60, 120) -> (-60, 80)
  line L43 (-64, 120) -> (-64, 80)
  line L44 (-64, 80) -> (-62, 80)
  line L45 (-62, 80) -> (-62, 120)
  line L46 (-62, 80) -> (-60, 80)
  line L47 (-56, 120) -> (-56, 80)
  line L48 (-58, 120) -> (-60, 120)
  line L49 (-62, 120) -> (-64, 120)
  line L50 (-52, 120) -> (-54, 120)
  line L51 (-54, 120) -> (-54, 80)
  line L52 (-54, 80) -> (-52, 80)
  line L53 (-52, 80) -> (-52, 120)
  line L54 (-40, 101.048831) -> (-75.000001, 101.048831)
  line L55 (-75.000001, 101.048831) -> (-75.000001, 99.000001)
  line L56 (-75.000001, 99.000001) -> (-40, 99.000001)
  line L57 (-40, 99.000001) -> (-40, 101.048831)
  line L58 (-72, 120) -> (-72, 80)
  line L59 (-74, 80) -> (-72, 80)
  line L60 (-68, 120) -> (-68, 80)
  line L61 (-66, 120) -> (-68, 120)
  line L62 (-78, 80) -> (-76, 80)
  line L63 (-74, 120) -> (-74, 80)
  line L64 (-76, 80) -> (-74, 80)
  line L65 (-74, 80) -> (-74, 120)
  line L66 (-70, 80) -> (-70, 120)
  line L67 (-66, 120) -> (-66, 80)
  line L68 (-78, 120) -> (-78, 80)
  line L69 (-68, 80) -> (-66, 80)
  line L70 (-66, 80) -> (-66, 120)
  line L71 (-72, 80) -> (-70, 80)
  line L72 (-68, 80) -> (-68, 120)
  line L73 (-76, 80) -> (-76, 120)
  line L74 (-70, 80) -> (-68, 80)
  line L75 (-72, 80) -> (-72, 120)
  line L76 (-76, 120) -> (-76, 80)
  line L77 (-70, 120) -> (-70, 80)
  line L78 (-76, 120) -> (-76, 80)
  line L79 (-68, 120) -> (-78, 120)
  dimension "d133" = 2
  dimension "d134" = 40
  dimension "d135" = 2
  dimension "d136" = 2
  dimension "d137" = 40
  dimension "d138" = 2
  dimension "d139" = 2
  dimension "d140" = 2
  dimension "d141" = 40
  dimension "d142" = 2
  dimension "d143" = 2
  dimension "d144" = 40
  dimension "d145" = 2
  dimension "d146" = 2
  dimension "d147" = 2
  dimension "d148" = 40
  dimension "d149" = 2
  dimension "d150" = 2
  dimension "d151" = 40
  dimension "d152" = 2
  dimension "d153" = 2
  constraint horizontal L0
  constraint vertical L1
  constraint horizontal L2
  constraint vertical L3
  constraint horizontal L4
  constraint vertical L5
  constraint horizontal L6
  constraint vertical L7
  constraint horizontal L8
  constraint vertical L9
  constraint horizontal L10
  constraint vertical L11
  constraint horizontal L12
  constraint vertical L13
  constraint horizontal L14
  constraint vertical L15
  constraint horizontal L17
  constraint vertical L18
  constraint horizontal L19
  constraint vertical L20
  constraint horizontal L21
  constraint vertical L22
  constraint horizontal L23
  constraint vertical L24
  constraint horizontal L30
  constraint vertical L47
  constraint horizontal L37
  constraint vertical L34
  constraint horizontal L31
  constraint vertical L40
  constraint horizontal L38
  constraint vertical L28
  constraint horizontal L48
  constraint vertical L42
  constraint horizontal L39
  constraint vertical L25
  constraint horizontal L32
  constraint vertical L41
  constraint horizontal L46
  constraint vertical L27
  constraint horizontal L35
  constraint vertical L33
  constraint horizontal L36
  constraint vertical L26
  constraint horizontal L49
  constraint vertical L43
  constraint horizontal L44
  constraint vertical L45
  constraint horizontal L50
  constraint vertical L51
  constraint horizontal L52
  constraint vertical L53
  constraint horizontal L54
  constraint vertical L55
  constraint horizontal L56
  constraint vertical L57
  constraint horizontal L61
  constraint vertical L60
  constraint horizontal L69
  constraint vertical L70
  constraint vertical L77
  constraint horizontal L74
  constraint vertical L72
  constraint vertical L58
  constraint horizontal L71
  constraint vertical L66
  constraint vertical L63
  constraint horizontal L59
  constraint vertical L75
  constraint vertical L68
  constraint horizontal L62
  constraint vertical L73
  constraint vertical L78
  constraint horizontal L64
  constraint vertical L65
  constraint vertical L67
  constraint perpendicular L68 L79
  measures "d133" distance of L0.start L0.end
  measures "d134" distance of L0.start L2.end
  measures "d135" distance of L0.end L4.end
  measures "d136" distance of L4.end L8.end
  measures "d137" distance of L4.end L5.end
  measures "d138" distance of L8.end L12.end
  measures "d139" distance of L16.start L17.end
  measures "d140" distance of L28.end L30.start
  measures "d141" distance of L30.start L34.start
  measures "d142" distance of L28.end L25.end
  measures "d143" distance of L25.end L27.end
  measures "d144" distance of L25.start L25.end
  measures "d145" distance of L32.end L27.end
  measures "d146" distance of L26.end L33.start
  measures "d147" distance of L33.start L60.start
  measures "d148" distance of L33.start L33.end
  measures "d149" distance of L66.end L60.start
  measures "d150" distance of L66.end L58.start
  measures "d151" distance of L66.end L66.start
  measures "d152" distance of L63.start L58.start
  measures "d153" distance of L73.end L68.start
extrude "Extrude27" cut sketch "Sketch31" against normal blind 10 contours L0 L1 L3 L7 L54 | L5 L8 L9 L11 L15 L54 | L1 L2 L3 L7 L56 | L5 L9 L10 L11 L15 L56 | L13 L16 L20 L21 L22 L24 L54 | L13 L16 L20 L22 L23 L24 L56 | L18 L34 L50 L51 L53 L54 | L18 L34 L51 L52 L53 L56 | L25 L28 L31 L40 L47 L54 | L25 L28 L38 L40 L47 L56 | L27 L32 L41 L42 L45 L54 | L27 L41 L42 L45 L46 L56 | L26 L29 L33 L35 L43 L54 L67 L70 | L26 L29 L33 L36 L43 L56 L67 L70 | L54 L60 L66 L72 L77 L79 | L56 L60 L66 L72 L74 L77 | L54 L58 L63 L65 L75 L79 | L56 L58 L59 L63 L65 L75 picked at (-41.333333, 113.682944) picked at (-45.333333, 113.682944) picked at (-41.333333, 92.666668) picked at (-44.666667, 86.333334) picked at (-49.333333, 113.682944) picked at (-49.333333, 92.666668) picked at (-53.333333, 113.682944) picked at (-53.333333, 92.666668) picked at (-57.333333, 113.682944) picked at (-57.333333, 92.666668) picked at (-60.666667, 107.365887) picked at (-61.333333, 92.666668) picked at (-65.333333, 113.682944) picked at (-65.333333, 92.666668) picked at (-69.333333, 113.682944) picked at (-69.333333, 92.666668) picked at (-73.333333, 113.682944) picked at (-73.333333, 92.666668) bodies 7
combine "Combine1" operation add target body 4 tool bodies 3 7 5 2 6
sketch "Sketch32" plane through (0, 0, 0) normal (1, 0, 0) x (0, 0, -1)
  line L0 (-10, -20) -> (-190, -20)
  line L1 (-190, -20) -> (-190, 300)
  line L2 (-190, 300) -> (-10, 300)
  line L3 (-10, 300) -> (-10, -20)
  constraint horizontal L0
  constraint vertical L1
  constraint horizontal L2
  constraint vertical L3
split "Split2" by curves path "Sketch32" along L2 L3 L0 L1 bodies 4 makes body 9 at (178.918149, 200, 180) makes body 10 at (178.918149, 200, 20) makes body 11 at (-178.918149, 200, 180) makes body 12 at (124.819691, 305, 95)
sketch "Sketch33" plane through (0, 0, 0) normal (0, 0, -1) x (-1, 0, 0)
  line L0 (-25.333333, 420) -> (-27.336546, 389.951807)
  line L1 (-27.336546, 389.951807) -> (-43.548602, 389.951807)
  line L2 (-43.548602, 389.951807) -> (-40.209914, 420)
  line L3 (-40.209914, 420) -> (-25.333333, 420)
  line L4 (59.111111, 420) -> (63.785274, 389.951807)
  line L5 (63.785274, 389.951807) -> (47.573218, 389.951807)
  line L6 (47.573218, 389.951807) -> (44.23453, 420)
  line L7 (44.23453, 420) -> (59.111111, 420)
  line L8 (48.017663, 385.951807) -> (64.407497, 385.951807)
  line L9 (64.407497, 385.951807) -> (70, 350)
  line L10 (70, 350) -> (52.012308, 350)
  line L11 (52.012308, 350) -> (48.017663, 385.951807)
  line L12 (-63.785274, 389.951807) -> (-59.111111, 420)
  line L13 (-59.111111, 420) -> (-44.23453, 420)
  line L14 (-44.23453, 420) -> (-47.573218, 389.951807)
  line L15 (-47.573218, 389.951807) -> (-63.785274, 389.951807)
  line L16 (-47.987692, 350) -> (-43.993047, 385.951807)
  line L17 (-43.993047, 385.951807) -> (-27.603213, 385.951807)
  line L18 (-27.603213, 385.951807) -> (-30, 350)
  line L19 (-30, 350) -> (-47.987692, 350)
  line L20 (40.209914, 420) -> (43.548602, 389.951807)
  line L21 (43.548602, 389.951807) -> (27.336546, 389.951807)
  line L22 (27.336546, 389.951807) -> (25.333333, 420)
  line L23 (25.333333, 420) -> (40.209914, 420)
  line L24 (43.993047, 385.951807) -> (47.987692, 350)
  line L25 (47.987692, 350) -> (30, 350)
  line L26 (30, 350) -> (27.603213, 385.951807)
  line L27 (27.603213, 385.951807) -> (43.993047, 385.951807)
  line L28 (-52.012308, 350) -> (-70, 350)
  line L29 (-70, 350) -> (-64.407497, 385.951807)
  line L30 (-64.407497, 385.951807) -> (-48.017663, 385.951807)
  line L31 (-48.017663, 385.951807) -> (-52.012308, 350)
  line L32 (263.504389, 9.486833) -> (116.666667, 450)
  line L33 (116.666667, 450) -> (-116.666667, 450)
  line L34 (-116.666667, 450) -> (-263.504389, 9.486833)
  arc A0 (-263.504389, 9.486833) -> (-235.04389, 0) centre (-249.27414, 4.743416) ccw
  line L35 (-235.04389, 0) -> (-135.04389, 300)
  line L36 (-135.04389, 300) -> (135.04389, 300)
  line L37 (135.04389, 300) -> (235.04389, 0)
  arc A1 (235.04389, 0) -> (263.504389, 9.486833) centre (249.27414, 4.743416) ccw
  line L38 (-235.04389, 0) -> (-263.504389, 9.486833)
  line L39 (-249.27414, 4.743416) -> (-254.576455, -9.486833)
  line L40 (-135.04389, 300) -> (-166.666667, 300)
  line L41 (-166.666667, 300, 0) -> (-166.666667, 300, -20)
  line L42 (-150.855278, 300) -> (-249.27414, 4.743416)
  line L43 (-154.650012, 301.264911) -> (-253.046784, 6.074594)
  line L44 (-253.046784, 6.074594) -> (-258.32471, -8.0902)
  line L45 (-147.060545, 298.735089) -> (-245.501495, 3.412239)
  line L46 (-245.501495, 3.412239) -> (-250.828199, -10.883466)
  line L47 (-147.060545, 298.735089) -> (-144.910548, 305.185081)
  point P0 (-166.666667, 300)
  dimension "d156" = 4
  dimension "d157" = -4
  constraint parallel L36 L40
  constraint parallel L45 L47
extrude "Extrude28" cut sketch "Sketch33" along normal blind -15 and the other way blind 5 contours L38 L40 L42 L43 L44 | L38 L40 L42 L45 L47 picked at (-185.067022, 201.581139) picked at (-182.396654, 201.159502) bodies 10 12
extrude "Extrude29" cut 1 faces at (182.396654, 201.159502, 5) along direction (0, 0, 1) blind 190 and the other way blind -180 on bodies 12 bodies 9 12